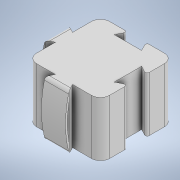
# Autodesk Inventor part: base
Saved by Autodesk Inventor 2022.2 (Build 262287010, 287A)
## iProperties
Part Number: base
Material: Generic
Document SubType Name: Modeling
Designer: yiunf
Appearance: Default
Author: yiunf
Autodesk Inventor part; units mm, degrees
ref_plane "YZ Plane" through (0, 0, 0) normal (1, 0, 0) x (0, 1, 0)
ref_plane "XZ Plane" through (0, 0, 0) normal (0, 1, 0) x (-1, 0, 0)
sketch "Sketch1" plane through (0, 0, 0) normal (0, 1, 0) x (-1, 0, 0)
  line L0 (-20, -20) -> (20, -20)
  line L1 (20, -20) -> (20, 20)
  line L2 (20, 20) -> (-20, 20)
  line L3 (-20, 20) -> (-20, -20)
  line L4 (-20, -20) -> (20, 20) construction
  line L5 (20, -20) -> (-20, 20) construction
  line L6 (20, 0) -> (20, 5)
  line L7 (20, 0) -> (25, 0)
  line L8 (25, 0) -> (25, 7.5)
  line L9 (25, 7.5) -> (20, 5)
  line L10 (25, 0) -> (25, -7.5)
  line L11 (20, 0) -> (20, -5)
  line L12 (20, -5) -> (25, -7.5)
  line L13 (0, 20) -> (5, 20)
  line L14 (0, 20) -> (0, 25)
  line L15 (0, 25) -> (7.5, 25)
  line L16 (7.5, 25) -> (5, 20)
  line L17 (0, 25) -> (-7.5, 25)
  line L18 (0, 20) -> (-5, 20)
  line L19 (-5, 20) -> (-7.5, 25)
  line L20 (0, -20) -> (5, -20)
  line L21 (7.5, -15) -> (5, -20)
  line L22 (0, -20) -> (-5, -20)
  line L23 (0, -20) -> (0, -15)
  line L24 (0, -15) -> (7.5, -15)
  line L25 (0, -15) -> (-7.5, -15)
  line L26 (-5, -20) -> (-7.5, -15)
  line L27 (-20, 0) -> (-20, 5)
  line L28 (-20, 0) -> (-20, -5)
  line L29 (-15, 0) -> (-15, -7.5)
  line L30 (-20, -5) -> (-15, -7.5)
  line L31 (-20, 0) -> (-15, 0)
  line L32 (-15, 7.5) -> (-20, 5)
  line L33 (-15, 0) -> (-15, 7.5)
  line L34 (24.75, 0) -> (24.75, 7.0955)
  line L35 (24.75, 7.0955) -> (20.25, 4.8455)
  line L36 (20.25, 4.8455) -> (20.25, 0)
  line L37 (24.75, 0) -> (24.75, -7.0955)
  line L38 (24.75, -7.0955) -> (20.25, -4.8455)
  line L39 (20.25, -4.8455) -> (20.25, 0)
  line L40 (0, 20.25) -> (4.8455, 20.25)
  line L41 (4.8455, 20.25) -> (7.0955, 24.75)
  line L42 (7.0955, 24.75) -> (0, 24.75)
  line L43 (0, 24.75) -> (-7.0955, 24.75)
  line L44 (-7.0955, 24.75) -> (-4.8455, 20.25)
  line L45 (-4.8455, 20.25) -> (0, 20.25)
  line L46 (24.75, 7.0955) -> (20, 4.7205)
  line L47 (24.75, -7.0955) -> (20, -4.7205)
  line L48 (7.0955, 24.75) -> (4.7205, 20)
  line L49 (-7.0955, 24.75) -> (-4.7205, 20)
  line L50 (25, 0) -> (23.75, 0)
  line L51 (23.75, 0) -> (23.75, 6.875)
  line L52 (23.75, 0) -> (23.75, -6.875)
  line L53 (0, 25) -> (0, 23.75)
  line L54 (0, 23.75) -> (6.875, 23.75)
  line L55 (0, 23.75) -> (-6.875, 23.75)
  point P0 (0, 0)
  point P1 (6.5955, 23.75)
  point P2 (-6.5955, 23.75)
  point P3 (23.75, -6.5955)
  point P4 (23.75, 6.5955)
  dimension "d0" = 40
  dimension "d1" = 40
  dimension "d2" = 5
  dimension "d3" = 5
  dimension "d4" = 7.5
  dimension "d5" = 7.5
  dimension "d6" = 5
  dimension "d9" = 40
  dimension "d16" = 40
  dimension "d21" = 0.25
  dimension "d22" = 0.25
  dimension "d23" = 0.25
  dimension "d24" = 0.25
  dimension "d29" = 1.25
  dimension "d30" = 1.25
  constraints: 112 end point, 21 point on line, 6 symmetric about line, 5 perpendicular, 3 horizontal, 3 midpoint, 2 parallel, 1 vertical, 34 other
  measures "d0" distance of L2.end L1.end
  measures "d1" distance of L1.end L0.end
  measures "d2" distance of L6.start L6.end
  measures "d3" distance of L6.start L7.end
  measures "d4" distance of L7.end L8.end
  measures "d5" distance of L7.end L10.end
  measures "d6" distance of L6.start L11.end
  measures "d9" distance of L13.end L20.end
  measures "d16" distance of L6.start L27.start
  measures "d21" distance between parallel lines of L8 L34
  measures "d22" distance between parallel lines of L10 L37
  measures "d23" distance between parallel lines of L16 L41
  measures "d24" distance between parallel lines of L17 L43
  measures "d29" distance of L7.end L50.end
  measures "d30" distance of L14.end L53.end
extrude "Extrusion1" add sketch "Sketch1" along normal blind 30 contours L3 L30 L29 L33 L32 L2 L1 L0 L21 L24 L25 L26 | L1 L7 L39 L47 | L49 L45 L14 L2 | L1 L46 L36 L7 | L39 L7 L52 L38 | L14 L40 L48 L2 | L44 L55 L14 L45 | L36 L35 L51 L7 | L14 L54 L41 L40
fillet "Fillet1" radius 5 4 edges at (20, 15, 20) (20, 15, -20) (-20, 15, -20) (-20, 15, 20)
fillet "Fillet2" radius 1 4 edges at (20, 15, 5) (20, 15, -5) (5, 15, -20) (-5, 15, -20)
ref_plane "Work Plane1" through (-6.5955, 0, 23.75) normal (1, 0, 0) x (0, 1, 0)
sketch "Sketch2" plane through (-6.5955, 0, 23.75) normal (1, 0, 0) x (0, 1, 0)
  line L0 (0, -3.75) -> (30, -3.75) projected
  line L1 (15, -3.75) -> (15, 2)
  line L2 (30, 0) -> (25, 0)
  line L3 (0, 0) -> (30, 0) projected
  line L4 (0, 0) -> (5, 0)
  arc A0 (30, 0) -> (0, 0) centre (15, -55.25) ccw
  line L5 (15, 2) -> (15, 1)
  arc A1 (25, 0) -> (5, 0) centre (15, -49.5) ccw
  point P0 (0, -23.75)
  dimension "d32" = 5.75
  dimension "d33" = 5
  dimension "d34" = 5
  dimension "d35" = 1
  constraints: 8 end point, 6 point on circle, 3 point on line, 2 centre point, 1 midpoint, 1 vertical
  measures "d32" distance of L1.start L1.end
  measures "d33" distance of L2.start L2.end
  measures "d34" distance of L3.start L4.end
  measures "d35" distance of L1.end L5.end
extrude "Extrusion2" add sketch "Sketch2" along normal blind 13.191 contours A1 L3 A0 L1 | L1 A0 L2 A1
fillet "Fillet3" radius 2 2 edges at (0, 30, 23.75) (0, 0, 23.75)
sketch "Sketch3" plane through (0, 30, 0) normal (0, 1, 0) x (1, 0, 0)
  point P0 (0, 0)
pattern_circular "Circular Pattern1" count 2 over 270 about axis through (0, 30, 0) along (0, 1, 0) of "Extrusion2", "Fillet3"
body "Solid1"
